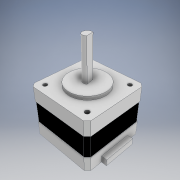
# Autodesk Inventor part: stepper
Saved by Autodesk Inventor 2020 (Build 240168000, 168)
## iProperties
Created: 2022-02-15
Part Number: stepper
Material: Generic
Document SubType Name: Modeling
Designer: Lars
Density: 1 g/cm^3
Appearance: Default
Author: Lars
Autodesk Inventor part; units mm, degrees
ref_plane "YZ Plane" through (0, 0, 0) normal (1, 0, 0) x (0, 1, 0)
ref_plane "XZ Plane" through (0, 0, 0) normal (0, 1, 0) x (-1, 0, 0)
ref_plane "XY Plane" through (0, 0, 0) normal (0, 0, 1) x (1, 0, 0)
sketch "Sketch1" plane through (0, 0, 0) normal (0, 1, 0) x (-1, 0, 0)
  line L0 (-15.5, -17.5) -> (15.5, -17.5)
  line L1 (17.5, -15.5) -> (17.5, 15.5)
  line L2 (15.5, 17.5) -> (-15.5, 17.5)
  line L3 (-17.5, 15.5) -> (-17.5, -15.5)
  line L4 (-17.5, -17.5) -> (17.5, 17.5) construction
  line L5 (17.5, -17.5) -> (-17.5, 17.5) construction
  line L6 (17.5, 15.5) -> (15.5, 17.5)
  line L7 (17.5, -15.5) -> (15.5, -17.5)
  line L8 (-15.5, -17.5) -> (-17.5, -15.5)
  line L9 (-15.5, 17.5) -> (-17.5, 15.5)
  point P0 (0, 0)
  dimension "d0" = 35
  dimension "d1" = 35
  dimension "d2" = 2
  dimension "d3" = 2
  dimension "d4" = 2
  dimension "d5" = 2
  dimension "d6" = 2
  dimension "d7" = 2
  dimension "d8" = 2
  dimension "d9" = 2
  constraints: 20 end point, 8 point on line, 2 midpoint, 2 parallel, 1 horizontal, 1 perpendicular
  measures "d0" distance of L5.start L4.end
  measures "d1" distance of L4.start L5.start
  measures "d2" distance of L1.end L4.end
  measures "d3" distance of L2.start L4.end
  measures "d4" distance of L1.start L5.start
  measures "d5" distance of L0.end L5.start
  measures "d6" distance of L0.start L4.start
  measures "d7" distance of L3.end L4.start
  measures "d8" distance of L2.end L5.end
  measures "d9" distance of L3.start L5.end
extrude "Extrusion1" add sketch "Sketch1" along normal blind 8
sketch "Sketch2" plane through (0, 8, 0) normal (0, 1, 0) x (1, 0, 0)
  line L0 (-17.5, -15.5) -> (-15.5, -17.5) projected
  line L1 (-15.5, -17.5) -> (15.5, -17.5) projected
  line L2 (15.5, -17.5) -> (17.5, -15.5) projected
  line L3 (17.5, -15.5) -> (17.5, 15.5) projected
  line L4 (17.5, 15.5) -> (15.5, 17.5) projected
  line L5 (15.5, 17.5) -> (-15.5, 17.5) projected
  line L6 (-15.5, 17.5) -> (-17.5, 15.5) projected
  line L7 (-17.5, 15.5) -> (-17.5, -15.5) projected
  line L8 (15.25, -17.25) -> (-15.25, -17.25)
  line L9 (-17.25, -15.25) -> (-17.25, 15.25)
  line L10 (-15.25, 17.25) -> (15.25, 17.25)
  line L11 (17.25, 15.25) -> (17.25, -15.25)
  line L12 (17.25, -17.25) -> (-17.25, 17.25) construction
  line L13 (-17.25, -17.25) -> (17.25, 17.25) construction
  line L14 (-17.25, 15.25) -> (-15.25, 17.25)
  line L15 (-17.25, -15.25) -> (-15.25, -17.25)
  line L16 (15.25, -17.25) -> (17.25, -15.25)
  line L17 (17.25, 15.25) -> (15.25, 17.25)
  point P0 (0, 0)
  dimension "d12" = 34.5
  dimension "d13" = 34.5
  dimension "d14" = 2
  dimension "d15" = 2
  dimension "d16" = 2
  dimension "d17" = 2
  dimension "d18" = 2
  dimension "d19" = 2
  dimension "d20" = 2
  dimension "d21" = 2
  constraints: 20 end point, 8 point on line, 2 midpoint, 2 parallel, 1 horizontal, 1 perpendicular
  measures "d12" distance of L12.end L13.end
  measures "d13" distance of L13.start L12.end
  measures "d14" distance of L9.end L12.end
  measures "d15" distance of L10.start L12.end
  measures "d16" distance of L9.start L13.start
  measures "d17" distance of L8.end L13.start
  measures "d18" distance of L8.start L12.start
  measures "d19" distance of L11.end L12.start
  measures "d20" distance of L11.start L13.end
  measures "d21" distance of L10.end L13.end
extrude "Extrusion2" add sketch "Sketch2" along normal blind 12 contours L8 L15 L9 L14 L10 L17 L11 L16
sketch "Sketch3" plane through (0, 20, 0) normal (0, 1, 0) x (1, 0, 0)
  line L0 (-17.5, -15.5) -> (-15.5, -17.5) projected
  line L1 (-17.5, 15.5) -> (-17.5, -15.5) projected
  line L2 (-15.5, 17.5) -> (-17.5, 15.5) projected
  line L3 (15.5, 17.5) -> (-15.5, 17.5) projected
  line L4 (17.5, 15.5) -> (15.5, 17.5) projected
  line L5 (17.5, -15.5) -> (17.5, 15.5) projected
  line L6 (15.5, -17.5) -> (17.5, -15.5) projected
  line L7 (-15.5, -17.5) -> (15.5, -17.5) projected
  point P0 (0, 0)
extrude "Extrusion3" add sketch "Sketch3" along normal blind 8
sketch "Sketch4" plane through (0, 28, 0) normal (0, 1, 0) x (1, 0, 0)
  circle A0 centre (0, 0) radius 11
  dimension "d26" = 22
  constraints: 1 centre point, 1 coincident
  measures "d26" diameter of A0
extrude "Extrusion4" add sketch "Sketch4" along normal blind 2
sketch "Sketch5" plane through (0, 30, 0) normal (0, 1, 0) x (1, 0, 0)
  arc A0 (0.7737, 2.3773) -> (1.6586, -1.8706) centre (0, 0) ccw
  line L0 (1.6586, -1.8706) -> (0.7737, 2.3773)
  dimension "d29" = 5
  constraints: 2 end point, 2 point on circle, 1 centre point, 1 coincident
  measures "d29" diameter of A0
extrude "Extrusion5" add sketch "Sketch5" along normal blind 22
sketch "Sketch6" plane through (0, 28, 0) normal (0, 1, 0) x (1, 0, 0)
  line L0 (15.5, 17.5) -> (-15.5, 17.5) projected
  line L1 (-17.5, 15.5) -> (-17.5, -15.5) projected
  line L2 (17.5, -15.5) -> (17.5, 15.5) projected
  line L3 (-15.5, -17.5) -> (15.5, -17.5) projected
  point P0 (0, 0)
  point P1 (-13, -13)
  point P2 (-13, 13)
  point P3 (13, 13)
  point P4 (13, -13)
  dimension "d32" = 26
  dimension "d33" = 26
  dimension "d34" = 4.5
  dimension "d35" = 4.5
  dimension "d45" = 4.5
  dimension "d46" = 4.5
  dimension "d47" = 4.5
  dimension "d48" = 4.5
  dimension "d49" = 4.5
  measures "d32" distance of point (-13, 13) point (-13, -13)
  measures "d33" distance of point (-13, 13) point (13, 13)
  measures "d34" distance from line of L0 point (-13, 13)
  measures "d35" distance from line of L1 point (-13, 13)
  measures "d45" distance from line of L1 point (-13, -13)
  measures "d46" distance from line of L2 point (13, -13)
  measures "d47" distance from line of L3 point (-13, -13)
  measures "d48" distance from line of L3 point (13, -13)
  measures "d49" distance from line of L0 point (13, 13)
hole "Hole1" at (-13, 28, 13) at (-13, 28, -13) at (13, 28, -13) at (13, 28, 13) direction (0, -1, 0) diameter 2.459 depth 8.8 tip angle 118 thread size "M3x0.5" class "6H" standard "ISO Metric profile"
sketch "Sketch7" plane through (17.5, 0, 15.5) normal (1, 0, 0) x (0, 0, -1)
  line L0 (31, 0) -> (0, 0) projected
  line L1 (24.2568, 0) -> (6.5267, 0)
  line L2 (6.5267, 0) -> (6.5267, 3.8069)
  line L3 (6.5267, 3.8069) -> (24.2568, 3.8069)
  line L4 (24.2568, 3.8069) -> (24.2568, 0)
  point P0 (15.5, 0)
  point P1 (6.5267, 0)
  constraints: 8 end point, 2 parallel, 1 horizontal, 1 perpendicular, 1 point on line
extrude "Extrusion6" add sketch "Sketch7" along normal blind 3
equation "\"d3\" = d2"
equation "\"d4\" = d2"
equation "\"d5\" = d4"
equation "\"d6\" = d2"
equation "\"d7\" = d6"
equation "\"d8\" = d2"
equation "\"d9\" = d8"
equation "\"d15\" = d14"
equation "\"d16\" = d14"
equation "\"d17\" = d16"
equation "\"d18\" = d14"
equation "\"d19\" = d18"
equation "\"d20\" = d14"
equation "\"d21\" = d20"
body "Solid1"
